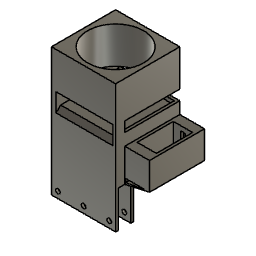
Sjoelbak (Autodesk Fusion 360 design; units mm, degrees)
Autodesk Fusion 360 part; units mm, degrees
sketch "Sketch1" plane through (0, 0, 0) normal (0, 0, 1) x (1, 0, 0)
  line L0 (0, 0) -> (70, 0)
  line L1 (70, 0) -> (70, -70)
  line L2 (70, -70) -> (0, -70)
  line L3 (0, -70) -> (0, 0)
  dimension "d3" = 70
  dimension "d4" = 70
  constraint horizontal L0
  constraint vertical L1
  constraint horizontal L2
  constraint vertical L3
  constraint coincident L0.start L3.end
  measures "d3" distance of L0.start L0.end
  measures "d4" distance of L0.start L2.end
extrude "Extrude1" add sketch "Sketch1" against normal blind 140
sketch "Sketch2" plane through (0, 0, 0) normal (0, 0, 1) x (-1, 0, 0)
  line L0 (0, 70) -> (-70, 70)
  line L1 (-70, 70) -> (-70, 0)
  line L2 (-70, 0) -> (0, 0)
  line L3 (0, 0) -> (0, 70)
  line L4 (0, 0) -> (-35, 0) construction
  line L5 (-35, 0) -> (-35, 35) construction
  circle A0 centre (-35, 35) radius 30.5
  dimension "d7" = 35
  dimension "d8" = 35
  dimension "d9" = 61
  constraint coincident L2.end L3.start
  constraint midpoint L2 L4.end
  constraint perpendicular L2 L5
  constraint coincident L5.end A0.centre
  measures "d7" distance of L2.end L4.end
  measures "d8" distance of L4.end L5.end
  measures "d9" diameter of A0
extrude "Extrude2" cut sketch "Sketch2" against normal blind 40 contours A0
sketch "Sketch3" plane through (0, -70, 0) normal (0, -1, 0) x (1, 0, 0)
  line L0 (70, 0) -> (0, 0)
  line L1 (0, 0) -> (0, -140)
  line L2 (0, -140) -> (70, -140)
  line L3 (70, -140) -> (70, 0)
  line L4 (0, 0) -> (0, -40) construction
  line L5 (0, -40) -> (5, -40) construction
  line L6 (5, -40) -> (5, -55) construction
  line L7 (5, -55) -> (70, -55)
  line L8 (70, -55) -> (70, -40)
  line L9 (70, -40) -> (5, -40)
  line L10 (5, -40) -> (5, -55)
  dimension "d12" = 40
  dimension "d13" = 5
  dimension "d14" = 15
  constraint coincident L0.end L1.start
  constraint perpendicular L0 L4
  constraint perpendicular L4 L5
  constraint perpendicular L5 L6
  constraint horizontal L7
  constraint vertical L8
  constraint horizontal L9
  constraint vertical L10
  constraint coincident L3 L8.end
  measures "d12" distance of L0.end L4.end
  measures "d13" distance of L4.end L5.end
  measures "d14" distance of L5.end L6.end
extrude "Extrude3" cut sketch "Sketch3" against normal blind 120 contours L3 L7 L8 L9 L10
sketch "Sketch4" plane through (70, 0, 0) normal (1, 0, 0) x (0, 1, 0)
  line L0 (0, -55) -> (-70, -55)
  line L1 (-70, -55) -> (-70, -140)
  line L2 (-70, -140) -> (0, -140)
  line L3 (0, -140) -> (0, -55)
  line L4 (-70, -140) -> (-67, -140) construction
  line L5 (-67, -140) -> (-53.5, -140)
  line L6 (-53.5, -140) -> (-53.5, -100)
  line L7 (-53.5, -100) -> (-67, -100)
  line L8 (-67, -100) -> (-67, -140)
  line L9 (-53.5, -140) -> (-50.5, -140) construction
  line L10 (-50.5, -140) -> (0, -140)
  line L11 (0, -140) -> (0, -100)
  line L12 (0, -100) -> (-50.5, -100)
  line L13 (-50.5, -100) -> (-50.5, -140)
  dimension "d19" = 3
  dimension "d20" = 13.5
  dimension "d21" = 40
  dimension "d24" = 3
  constraint coincident L1.end L2.start
  constraint perpendicular L1 L4
  constraint horizontal L5
  constraint vertical L6
  constraint horizontal L7
  constraint vertical L8
  constraint perpendicular L6 L9
  constraint horizontal L10
  constraint vertical L11
  constraint horizontal L12
  constraint vertical L13
  constraint coincident L3 L11.end
  measures "d19" distance of L1.end L4.end
  measures "d20" distance of L4.end L5.end
  measures "d21" distance of L4.end L7.end
  measures "d24" distance of L5.end L9.end
extrude "Extrude4" cut sketch "Sketch4" against normal blind 170 contours L2 L3 L10 L11 L12 L13 | L2 L5 L6 L7 L8
sketch "Sketch5" plane through (0, 0, 0) normal (0, 1, 0) x (-1, 0, 0)
  line L0 (-70, -100) -> (0, -100)
  line L1 (0, -100) -> (0, 0)
  line L2 (0, 0) -> (-70, 0)
  line L3 (-70, -40) -> (-5, -40)
  line L4 (-5, -40) -> (-5, -55)
  line L5 (-5, -55) -> (-70, -55)
  line L6 (-70, 0) -> (-70, -40)
  line L7 (-70, -100) -> (-67, -100)
  line L8 (-67, -100) -> (0, -100)
  line L9 (0, -100) -> (0, -65)
  line L10 (0, -65) -> (-67, -65)
  line L11 (-67, -65) -> (-67, -100)
  line L12 (-70, -55) -> (-70, -100)
  dimension "d25" = 3
  dimension "d26" = 67
  dimension "d27" = 35
  constraint coincident L0.start L7.start
  constraint perpendicular L6 L7
  constraint horizontal L8
  constraint vertical L9
  constraint horizontal L10
  constraint vertical L11
  measures "d25" distance of L0.start L7.end
  measures "d26" distance of L7.end L0.end
  measures "d27" distance of L7.end L10.end
extrude "Extrude5" cut sketch "Sketch5" against normal blind 50.5 contours L0 L1 L8 L9 L10 L11
sketch "Sketch6" plane through (0, 0, 0) normal (-1, 0, 0) x (0, -1, 0)
  line L0 (50.5, -65) -> (50.5, -140)
  line L1 (50.5, -140) -> (53.5, -140)
  line L2 (53.5, -140) -> (53.5, -100)
  line L3 (53.5, -100) -> (67, -100)
  line L4 (67, -100) -> (67, -140)
  line L5 (67, -140) -> (70, -140)
  line L6 (70, -140) -> (70, 0)
  line L7 (70, 0) -> (0, 0)
  line L8 (0, 0) -> (0, -65)
  line L9 (0, -65) -> (50.5, -65)
  line L10 (0, -65) -> (50.5, -100)
  line L11 (50.5, -100) -> (50.5, -95)
  line L12 (0, -65) -> (5, -65)
  line L13 (5, -65) -> (50.5, -95)
  constraint coincident L8.end L9.start
  constraint coincident L0 L10.end
  constraint coincident L0 L11.end
  constraint perpendicular L3 L11
  constraint coincident L9 L12.end
  constraint perpendicular L8 L12
extrude "Extrude6" add sketch "Sketch6" against normal blind 10 contours L0 L9 L10 L11 L12 L13
sketch "Sketch8" plane through (0, 0, 0) normal (-1, 0, 0) x (0, -1, 0)
  line L0 (50.5, -100) -> (50.5, -140)
  line L1 (50.5, -140) -> (53.5, -140)
  line L2 (53.5, -140) -> (53.5, -100)
  line L3 (53.5, -100) -> (67, -100)
  line L4 (67, -100) -> (67, -140)
  line L5 (67, -140) -> (70, -140)
  line L6 (70, -140) -> (70, 0)
  line L7 (70, 0) -> (0, 0)
  line L8 (0, 0) -> (0, -65)
  line L9 (0, -65) -> (50.5, -100)
  line L10 (50.5, -95) -> (5, -65)
  line L11 (5, -65) -> (50.5, -65)
  line L12 (50.5, -65) -> (50.5, -95)
  line L13 (27.75, -80) -> (29.8372, -81.3761)
  line L14 (50.5, -65) -> (50.5, -67.5)
  line L15 (29.8372, -81.3761) -> (50.5, -67.5)
  line L16 (27.75, -80) -> (25.6628, -78.6239)
  line L17 (50.5, -65) -> (48, -65)
  line L18 (25.6628, -78.6239) -> (48, -65)
  dimension "d35" = 2.5
  dimension "d36" = 2.5
  dimension "d37" = 2.5
  dimension "d38" = 2.5
  constraint coincident L11.end L12.start
  constraint midpoint L10 L13.start
  constraint parallel L10 L13
  constraint perpendicular L11 L14
  constraint parallel L10 L16
  constraint perpendicular L14 L17
  measures "d35" distance of L13.start L13.end
  measures "d36" distance of L11.end L14.end
  measures "d37" distance of L13.start L16.end
  measures "d38" distance of L11.end L17.end
extrude "Extrude7" add sketch "Sketch8" against normal blind 10 contours L10 L11 L12 L13 L14 L15 L16 L17 L18
fillet "Fillet2" radius 1.5 6 edges at (5, -25.6628, -78.6239) (5, -50.5, -95) (5, -50.5, -67.5) (5, -29.8372, -81.3761) (5, -5, -65) (5, -48, -65)
sketch "Sketch10" plane through (0, -70, 0) normal (0, -1, 0) x (1, 0, 0)
  line L0 (70, 0) -> (0, 0)
  line L1 (0, 0) -> (0, -140)
  line L2 (0, -140) -> (70, -140)
  line L3 (70, -40) -> (70, 0)
  line L4 (70, -55) -> (5, -55)
  line L5 (5, -55) -> (5, -40)
  line L6 (5, -40) -> (70, -40)
  line L7 (0, -140) -> (0, -133) construction
  line L8 (0, -133) -> (7, -133) construction
  line L9 (70, -40) -> (70, -33) construction
  line L10 (70, -33) -> (63, -33) construction
  circle A0 centre (7, -133) radius 2.5
  circle A1 centre (35, -133) radius 2.5
  circle A2 centre (63, -133) radius 2.5
  line L11 (70, -140) -> (70, -55)
  dimension "d43" = 7
  dimension "d44" = 7
  dimension "d45" = 7
  dimension "d46" = 7
  dimension "d47" = 5
  dimension "d50" = 56
  dimension "d51" = 0
  constraint coincident L1.end L2.start
  constraint perpendicular L2 L7
  constraint perpendicular L7 L8
  constraint coincident L3.start L6.end
  constraint perpendicular L2 L9
  constraint perpendicular L9 L10
  constraint coincident L8.end A0.centre
  measures "d43" distance of L1.end L7.end
  measures "d44" distance of L7.end L8.end
  measures "d45" distance of L3.start L9.end
  measures "d46" distance of L9.end L10.end
  measures "d47" diameter of A0
extrude "Extrude8" cut sketch "Sketch10" against normal blind 30 contours A0 | A1 | A2
chamfer "Chamfer1" distance 5 angle 45 1 edges at (37.5, -70, -55)
sketch "Sketch11" plane through (0, 0, -55) normal (0, 0, 1) x (-1, 0, 0)
  line L0 (-5, 65) -> (-70, 65)
  line L1 (-70, 65) -> (-70, 0)
  line L2 (-70, 0) -> (-5, 0)
  line L3 (-5, 0) -> (-5, 65)
  line L4 (-70, 70) -> (-67, 70)
  line L5 (-67, 70) -> (-67, 0)
  line L6 (-67, 0) -> (-70, 0)
  line L7 (-70, 0) -> (-70, 70)
  dimension "d55" = 3
  dimension "d56" = 70
  constraint horizontal L4
  constraint vertical L5
  constraint horizontal L6
  constraint vertical L7
  measures "d55" distance of L4.start L4.end
  measures "d56" distance of L4.start L1.end
extrude "Extrude9" add sketch "Sketch11" along normal blind 4 contours L0 L1 L2 L5 L6 L7 | L0 L4 L5 L7
extrude "Extrude10" add 1 faces at (69, -68.3333, -55) along direction (0, 0, -1) up to surface end surface through (5, -67.5, -57.5) normal (0, -0.707107, 0.707107) offset 0
sketch "Sketch12" plane through (67, 0, 0) normal (-1, 0, 0) x (0, -1, 0)
  line L0 (70, -60) -> (70, -51)
  line L1 (70, -51) -> (0, -51)
  line L2 (0, -51) -> (0, -55)
  line L3 (0, -55) -> (65, -55)
  line L4 (65, -55) -> (70, -60)
  line L5 (0, -51) -> (3, -51)
  line L6 (3, -51) -> (3, -55)
  line L7 (3, -55) -> (0, -55)
  line L8 (0, -55) -> (0, -51)
  dimension "d61" = 3
  dimension "d62" = 4
  constraint horizontal L5
  constraint vertical L6
  constraint horizontal L7
  constraint vertical L8
  constraint coincident L1.end L2.start
  measures "d61" distance of L1.end L5.end
  measures "d62" distance of L1.end L2.end
extrude "Extrude11" add sketch "Sketch12" along normal up to surface (62 mm away) contours L1 L2 L3 L5 L6 L7 L8
sketch "Sketch13" plane through (0, 0, -51) normal (0, 0, 1) x (-1, 0, 0)
  line L0 (-70, 0) -> (-5, 0)
  line L1 (-5, 0) -> (-5, 3)
  line L2 (-5, 3) -> (-67, 3)
  line L3 (-67, 3) -> (-67, 70)
  line L4 (-67, 70) -> (-70, 70)
  line L5 (-70, 70) -> (-70, 0)
  line L6 (-67, 70) -> (-70, 70)
  line L7 (-70, 70) -> (-70, 60)
  line L8 (-70, 60) -> (-67, 60)
  line L9 (-67, 60) -> (-67, 70)
  dimension "d65" = 3
  dimension "d66" = 10
  constraint horizontal L6
  constraint vertical L7
  constraint horizontal L8
  constraint vertical L9
  constraint coincident L3.end L4.start
  measures "d65" distance of L3.end L4.end
  measures "d66" distance of L3.end L8.end
extrude "Extrude12" add sketch "Sketch13" along normal up to surface (11 mm away) contours L3 L4 L5 L6 L7 L8 L9
sketch "Sketch14" plane through (70, 0, 0) normal (1, 0, 0) x (0, 1, 0)
  line L0 (-70, 0) -> (-70, -140)
  line L1 (-70, -140) -> (-67, -140)
  line L2 (-67, -140) -> (-67, -100)
  line L3 (-67, -100) -> (-53.5, -100)
  line L4 (-53.5, -100) -> (-53.5, -140)
  line L5 (-53.5, -140) -> (-50.5, -140)
  line L6 (-50.5, -140) -> (-50.5, -100)
  line L7 (-50.5, -100) -> (0, -100)
  line L8 (0, -100) -> (0, -51)
  line L9 (0, -51) -> (-60, -51)
  line L10 (-60, -51) -> (-60, -40)
  line L11 (-60, -40) -> (0, -40)
  line L12 (0, -40) -> (0, 0)
  line L13 (0, 0) -> (-70, 0)
  line L14 (0, -51) -> (0, -64) construction
  line L15 (0, -64) -> (-60, -64)
  line L16 (-60, -64) -> (-60, -94)
  line L17 (-60, -94) -> (0, -94)
  line L18 (0, -94) -> (0, -64)
  dimension "d69" = 13
  dimension "d70" = 60
  dimension "d71" = 30
  constraint coincident L8.end L9.start
  constraint perpendicular L9 L14
  constraint horizontal L15
  constraint vertical L16
  constraint horizontal L17
  constraint vertical L18
  measures "d69" distance of L8.end L14.end
  measures "d70" distance of L14.end L15.end
  measures "d71" distance of L14.end L17.end
extrude "Extrude13" add sketch "Sketch14" along normal blind 27 contours L8 L15 L16 L17 L18
sketch "Sketch15" plane through (0, 0, -64) normal (0, 0, 1) x (-1, 0, 0)
  line L0 (-70, 0) -> (-70, 60)
  line L1 (-70, 60) -> (-97, 60)
  line L2 (-97, 60) -> (-97, 0)
  line L3 (-97, 0) -> (-70, 0)
  line L4 (-97, 0) -> (-97, 10) construction
  line L5 (-97, 60) -> (-97, 49.5) construction
  line L6 (-70, 60) -> (-70, 49.5) construction
  line L7 (-70, 0) -> (-70, 10) construction
  line L8 (-70, 49.5) -> (-73, 49.5) construction
  line L9 (-97, 10) -> (-94, 10) construction
  line L10 (-73, 49.5) -> (-94, 49.5)
  line L11 (-94, 49.5) -> (-94, 10)
  line L12 (-94, 10) -> (-73, 10)
  line L13 (-73, 10) -> (-73, 49.5)
  dimension "d74" = 10
  dimension "d75" = 10.5
  dimension "d76" = 10.5
  dimension "d77" = 10
  dimension "d78" = 3
  dimension "d79" = 3
  constraint coincident L2.end L3.start
  constraint perpendicular L3 L4
  constraint coincident L1.end L2.start
  constraint perpendicular L1 L5
  constraint coincident L0.end L1.start
  constraint perpendicular L1 L6
  constraint coincident L0.start L3.end
  constraint perpendicular L3 L7
  constraint perpendicular L6 L8
  constraint perpendicular L2 L9
  constraint horizontal L10
  constraint vertical L11
  constraint horizontal L12
  constraint vertical L13
  measures "d74" distance of L2.end L4.end
  measures "d75" distance of L1.end L5.end
  measures "d76" distance of L0.end L6.end
  measures "d77" distance of L0.start L7.end
  measures "d78" distance of L6.end L8.end
  measures "d79" distance of L4.end L9.end
extrude "Extrude14" cut sketch "Sketch15" against normal blind 36 contours L10 L11 L12 L13
sketch "Sketch16" plane through (0, 0, 0) normal (0, 1, 0) x (-1, 0, 0)
  line L0 (-67, -65) -> (-10, -65)
  line L1 (-10, -65) -> (0, -65)
  line L2 (0, -65) -> (0, 0)
  line L3 (0, 0) -> (-70, 0)
  line L4 (-70, 0) -> (-70, -40)
  line L5 (-70, -40) -> (-5, -40)
  line L6 (-5, -40) -> (-5, -51)
  line L7 (-5, -51) -> (-70, -51)
  line L8 (-70, -51) -> (-70, -64)
  line L9 (-70, -64) -> (-97, -64)
  line L10 (-97, -64) -> (-97, -94)
  line L11 (-97, -94) -> (-70, -94)
  line L12 (-70, -94) -> (-70, -100)
  line L13 (-70, -100) -> (-67, -100)
  line L14 (-67, -100) -> (-67, -65)
  line L15 (-97, -94) -> (-70, -100)
  line L16 (-70, -100) -> (-70, -98)
  line L17 (-97, -94) -> (-95, -94)
  line L18 (-95, -94) -> (-92.5, -94)
  line L19 (-92.5, -94) -> (-70, -98)
  line L20 (-95.8, -95.2) -> (-95.7872, -95.1423)
  dimension "d82" = 2
  dimension "d83" = 2
  constraint coincident L10.end L11.start
  constraint coincident L12.end L13.start
  constraint perpendicular L13 L16
  constraint perpendicular L10 L17
  constraint coincident L11 L18.end
  constraint perpendicular L16 L18
  constraint perpendicular L15 L20
  measures "d82" distance of L12.end L16.end
  measures "d83" distance of L10.end L17.end
extrude "Extrude15" add sketch "Sketch16" against normal blind 5 contours L11 L12 L15 L16 L17 L18 L19
sketch "Sketch17" plane through (0, -60, 0) normal (0, -1, 0) x (1, 0, 0)
  line L0 (70, -64) -> (70, -94)
  line L1 (70, -94) -> (97, -94)
  line L2 (97, -94) -> (97, -64)
  line L3 (97, -64) -> (70, -64)
  line L4 (70, -94) -> (70, -100) construction
  line L5 (70, -100) -> (70, -98)
  line L6 (97, -94) -> (93, -94)
  line L7 (70, -100) -> (97, -94)
  line L8 (93, -94) -> (70, -98)
  dimension "d86" = 2
  dimension "d87" = 4
  constraint coincident L0.end L1.start
  constraint perpendicular L1 L4
  constraint perpendicular L1 L5
  constraint coincident L1.end L2.start
  constraint perpendicular L2 L6
  measures "d86" distance of L4.end L5.end
  measures "d87" distance of L1.end L6.end
extrude "Extrude16" add sketch "Sketch17" against normal blind 5 contours L1 L5 L6 L7 L8
sketch "Sketch18" plane through (0, 0, -94) normal (0, 0, -1) x (1, 0, 0)
  line L0 (73, 49.5) -> (94, 49.5)
  line L1 (94, 49.5) -> (94, 10)
  line L2 (94, 10) -> (73, 10)
  line L3 (73, 10) -> (73, 49.5)
  line L4 (97, 55) -> (93, 55)
  line L5 (93, 55) -> (93, 60)
  line L6 (93, 60) -> (70, 60)
  line L7 (70, 60) -> (70, 0)
  line L8 (70, 0) -> (92.5, 0)
  line L9 (92.5, 0) -> (92.5, 5)
  line L10 (92.5, 5) -> (97, 5)
  line L11 (97, 5) -> (97, 55)
  line L12 (73, 10) -> (94, 10) construction
  line L13 (83.5, 10) -> (86, 10)
  line L14 (86, 10) -> (81, 10)
  line L15 (81, 10) -> (81, 7)
  line L16 (81, 7) -> (86, 7)
  line L17 (86, 7) -> (86, 10)
  dimension "d90" = 2.5
  dimension "d91" = 3
  constraint coincident L2.end L3.start
  constraint coincident L1.end L2.start
  constraint midpoint L12 L13.start
  constraint parallel L12 L13
  constraint horizontal L14
  constraint vertical L15
  constraint horizontal L16
  constraint vertical L17
  measures "d90" distance of L13.start L13.end
  measures "d91" distance of L13.end L16.end
extrude "Extrude17" cut sketch "Sketch18" against normal blind 25 contours L2 L13 L14 L15 L16 L17
sketch "Sketch19" plane through (0, 0, -94) normal (0, 0, -1) x (1, 0, 0)
  line L0 (97, 55) -> (93, 55)
  line L1 (93, 55) -> (93, 60)
  line L2 (93, 60) -> (70, 60)
  line L3 (70, 60) -> (70, 0)
  line L4 (70, 0) -> (92.5, 0)
  line L5 (92.5, 0) -> (92.5, 5)
  line L6 (92.5, 5) -> (97, 5)
  line L7 (97, 5) -> (97, 55)
  line L8 (86, 10) -> (86, 7)
  line L9 (86, 7) -> (81, 7)
  line L10 (81, 7) -> (81, 10)
  line L11 (81, 10) -> (73, 10)
  line L12 (73, 10) -> (73, 49.5)
  line L13 (73, 49.5) -> (94, 49.5)
  line L14 (94, 49.5) -> (94, 10)
  line L15 (94, 10) -> (86, 10)
  line L16 (70, 60) -> (71, 60)
  line L17 (71, 60) -> (71, 55)
  line L18 (71, 55) -> (70, 55)
  line L19 (70, 55) -> (70, 60)
  line L20 (70, 0) -> (71, 0)
  line L21 (71, 0) -> (71, 5)
  line L22 (71, 5) -> (70, 5)
  line L23 (70, 5) -> (70, 0)
  dimension "d94" = 1
  dimension "d95" = 5
  dimension "d96" = 1
  dimension "d97" = 5
  constraint horizontal L16
  constraint vertical L17
  constraint horizontal L18
  constraint vertical L19
  constraint coincident L2.end L3.start
  constraint horizontal L20
  constraint vertical L21
  constraint horizontal L22
  constraint vertical L23
  constraint coincident L3.end L4.start
  measures "d94" distance of L2.end L16.end
  measures "d95" distance of L2.end L18.end
  measures "d96" distance of L3.end L20.end
  measures "d97" distance of L3.end L22.end
extrude "Extrude18" add sketch "Sketch19" along normal up to surface contours L2 L3 L16 L17 L18 L19 | L3 L4 L20 L21 L22 L23 end surface through (92.5, 0, -94) normal (-0.175033, 0, 0.984563) offset 0
fillet "Fillet3" radius 0.2 6 edges at (71, -2.5, -94) (71, -2.5, -97.8222) (92.5, -2.5, -94) (71, -57.5, -94) (71, -57.5, -97.8222) (93, -57.5, -94)
sketch "Sketch20" plane through (0, 0, -55) normal (0, 0, 1) x (-1, 0, 0)
  line L0 (-67, 3) -> (-5, 3)
  line L1 (-5, 3) -> (-5, 65)
  line L2 (-5, 65) -> (-67, 65)
  line L3 (-67, 65) -> (-67, 3)
  line L4 (-70, 0) -> (-35, 0) construction
  line L5 (-35, 0) -> (-35, 35) construction
  line L6 (-35, 35) -> (-35, 40) construction
  line L7 (-35, 35) -> (-35, 30) construction
  line L8 (-35, 40) -> (-27.5, 40) construction
  line L9 (-27.5, 40) -> (-42.5, 40)
  line L10 (-42.5, 40) -> (-42.5, 25)
  line L11 (-42.5, 25) -> (-27.5, 25)
  line L12 (-27.5, 25) -> (-27.5, 40)
  dimension "d102" = 35
  dimension "d103" = 35
  dimension "d104" = 5
  dimension "d105" = 5
  dimension "d107" = 7.5
  dimension "d108" = 15
  dimension "d109" = 15
  constraint parallel L0 L4
  constraint perpendicular L4 L5
  constraint parallel L5 L6
  constraint parallel L5 L7
  constraint perpendicular L6 L8
  constraint horizontal L9
  constraint vertical L10
  constraint horizontal L11
  constraint vertical L12
  measures "d102" distance of L4.start L4.end
  measures "d103" distance of L4.end L5.end
  measures "d104" distance of L5.end L6.end
  measures "d105" distance of L5.end L7.end
  measures "d107" distance of L6.end L8.end
  measures "d108" distance of L8.end L9.end
  measures "d109" distance of L8.end L11.end
extrude "Extrude19" cut sketch "Sketch20" against normal blind 1 contours L9 L10 L11 L12
sketch "Sketch21" plane through (0, 0, -56) normal (0, 0, 1) x (-1, 0, 0)
  line L0 (-27.5, 25) -> (-27.5, 40)
  line L1 (-27.5, 40) -> (-42.5, 40)
  line L2 (-42.5, 40) -> (-42.5, 25)
  line L3 (-42.5, 25) -> (-27.5, 25)
  line L4 (-42.5, 40) -> (-35, 40) construction
  line L5 (-35, 40) -> (-35, 38) construction
  circle A0 centre (-35, 35.5) radius 2.5
  line L6 (-34.9971, 33) -> (-34.9971, 31) construction
  circle A1 centre (-35.2251, 28.5104) radius 2.5
  dimension "d112" = 2
  dimension "d113" = 5
  dimension "d114" = 2
  dimension "d115" = 5
  constraint coincident L1.end L2.start
  constraint midpoint L1 L4.end
  constraint perpendicular L4 L5
  constraint coincident L5.end A0
  constraint coincident A0 L6.start
  constraint vertical L6
  constraint coincident L6.end A1
  measures "d112" distance of L4.end L5.end
  measures "d113" diameter of A0
  measures "d114" distance of L6.start L6.end
  measures "d115" diameter of A1
extrude "Extrude20" cut sketch "Sketch21" against normal blind 14 contours A0 | A1
sketch "Sketch22" plane through (0, 0, -65) normal (0, 0, -1) x (1, 0, 0)
  circle A0 centre (35, 35.5) radius 2.5
  circle A1 centre (35.2251, 28.5104) radius 2.5
  line L0 (10, 42.66) -> (0, 42.66)
  line L1 (0, 42.66) -> (0, 10)
  line L2 (0, 10) -> (10, 10)
  line L3 (10, 10) -> (10, 0)
  line L4 (10, 0) -> (67, 0)
  line L5 (67, 0) -> (67, 50.5)
  line L6 (67, 50.5) -> (10, 50.5)
  line L7 (10, 50.5) -> (10, 42.66)
  line L8 (35.2251, 26.0104) -> (35.2251, 24.0104) construction
  line L9 (34.9884, 38) -> (34.9884, 40) construction
  line L10 (35.2251, 24.0104) -> (27.4251, 24.0104) construction
  line L11 (27.4251, 24.0104) -> (42.4251, 24.0104)
  line L12 (42.4251, 24.0104) -> (42.4251, 40.0104)
  line L13 (42.4251, 40.0104) -> (27.4251, 40.0104)
  line L14 (27.4251, 40.0104) -> (27.4251, 24.0104)
  dimension "d118" = 2
  dimension "d119" = 2
  dimension "d120" = 7.8
  dimension "d121" = 15
  dimension "d122" = 16
  constraint coincident A1 L8.start
  constraint vertical L8
  constraint coincident A0 L9.start
  constraint vertical L9
  constraint perpendicular L8 L10
  constraint horizontal L11
  constraint vertical L12
  constraint horizontal L13
  constraint vertical L14
  measures "d118" distance of L8.start L8.end
  measures "d119" distance of L9.start L9.end
  measures "d120" distance of L8.end L10.end
  measures "d121" distance of L10.end L11.end
  measures "d122" distance of L10.end L13.end
extrude "Extrude21" cut sketch "Sketch22" against normal blind 7 contours L11 L12 L13 L14
